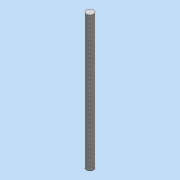
# Autodesk Inventor part: eje roscado
Saved by Autodesk Inventor 2017 (Build 210142000, 142)
## iProperties
Part Number: eje roscado
Material: Genérico
Document SubType Name: Modeling
Designer: Miguel A.
Density: 1 g/cm^3
Appearance: Valor por defecto
Author: Miguel A.
Autodesk Inventor part; units mm, degrees
ref_plane "YZ Plane" through (0, 0, 0) normal (1, 0, 0) x (0, 1, 0)
ref_plane "XZ Plane" through (0, 0, 0) normal (0, 1, 0) x (-1, 0, 0)
ref_plane "XY Plane" through (0, 0, 0) normal (0, 0, 1) x (1, 0, 0)
sketch "Boceto1" plane through (0, 0, 0) normal (0, 0, 1) x (1, 0, 0)
  circle A0 centre (0, 0) radius 4
  dimension "d0" = 8
  constraints: 1 centre point, 1 coincident
  measures "d0" diameter of A0
extrude "Extrusión1" add sketch "Boceto1" along normal mid plane 150
thread "Rosca1" size "M8x1.25" class "6g" standard "ISO Metric profile" full length
